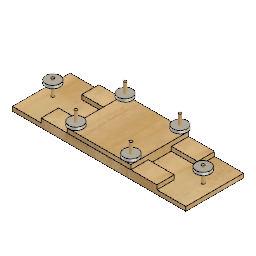
model_X (Autodesk Fusion 360 design; units mm, degrees)
Autodesk Fusion 360 part; units mm, degrees
sketch "Sketch1" plane through (0, 0, 0) normal (0, 0, 1) x (1, 0, 0)
  line L0 (300, 100) -> (-300, 100)
  line L1 (-300, 100) -> (-300, -100)
  line L2 (-300, -100) -> (300, -100)
  line L3 (300, -100) -> (300, 100)
  line L4 (300, 100) -> (-300, -100) construction
  line L5 (-300, 100) -> (300, -100) construction
  circle A0 centre (-260, 0) radius 5
  circle A1 centre (260, 0) radius 5
  line L6 (-200, -100) -> (200, -100)
  line L7 (200, -100) -> (200, -40)
  line L8 (200, -40) -> (-200, -40)
  line L9 (-200, -40) -> (-200, -100)
  line L10 (-200, 100) -> (200, 100)
  line L11 (200, 100) -> (200, 40)
  line L12 (200, 40) -> (-200, 40)
  line L13 (-200, 40) -> (-200, 100)
  circle A2 through (-235, 0, 55) (-272.5, 21.6506, 55) (-272.5, -21.6506, 55)
  circle A3 through (285, 0, 55) (247.5, 21.6506, 55) (247.5, -21.6506, 55)
  dimension "d1" = 600
  dimension "d2" = 200
  dimension "d3" = 40
  dimension "d4" = 40
  dimension "d5" = 10
  dimension "d6" = 10
  dimension "d7" = 400
  dimension "d8" = 60
  dimension "d9" = 400
  dimension "d10" = 60
  dimension "d11" = 100
  dimension "d12" = 100
  measures "d5" diameter of A0
  measures "d6" diameter of A1
  measures "d9" distance of L11 L13
  measures "d10" distance of L0 L12
  measures "d12" distance of L3 L7
extrude "Extrude1" add sketch "Sketch1" along normal blind 15 contours L0 L1 L2 L3 L7 L8 L9 L11 L12 L13 | L0 L10 L11 L12 L13 | L2 L6 L7 L8 L9 | A0 | A1 makes body 1
extrude "Extrude2" add sketch "Sketch1" along normal blind 30 contours L0 L10 L11 L12 L13 | L2 L6 L7 L8 L9 bodies 1
extrude "Extrude3" add sketch "Sketch1" along normal blind 70 contours A0 | A1 bodies 1
ref_plane "WorkPlane1" through (0, 0, 30) normal (0, 0, 1) x (1, 0, 0)
sketch "Sketch2" plane through (0, 0, 30) normal (0, 0, 1) x (1, 0, 0)
  line L0 (110, 39.5) -> (-110, 39.5)
  line L1 (-110, 39.5) -> (-110, -39.5)
  line L2 (-110, -39.5) -> (110, -39.5)
  line L3 (110, -39.5) -> (110, 39.5)
  line L4 (110, 39.5) -> (-110, -39.5) construction
  line L5 (-110, 39.5) -> (110, -39.5) construction
  line L6 (-110, 100) -> (110, 100)
  line L7 (110, 100) -> (110, -100)
  line L8 (110, -100) -> (-110, -100)
  line L9 (-110, -100) -> (-110, 100)
  line L10 (300, 100) -> (-300, 100)
  line L11 (-300, -100) -> (300, -100)
  circle A0 centre (-95, -85) radius 5
  circle A1 centre (95, -85) radius 5
  circle A2 centre (-95, 85) radius 5
  circle A3 centre (95, 85) radius 5
  circle A4 through (120, -85, 25) (82.5, -63.3494, 25) (82.5, -106.6506, 25)
  circle A5 through (-70, -85, 25) (-107.5, -63.3494, 25) (-107.5, -106.6506, 25)
  circle A6 through (-70, 85, 25) (-107.5, 106.6506, 25) (-107.5, 63.3494, 25)
  circle A7 through (120, 85, 25) (82.5, 106.6506, 25) (82.5, 63.3494, 25)
  line L12 (-70, -85) -> (-70, -100) construction
  line L13 (69.9377, -85) -> (70, -100) construction
  line L14 (70, 85) -> (70, 100) construction
  line L15 (-70, 85) -> (-70, 100) construction
  line L16 (70, -100) -> (60, -100) construction
  line L17 (-70, 100) -> (-60, 100) construction
  line L18 (-60, 100) -> (60, 100)
  line L19 (60, 100) -> (60, -100)
  line L20 (60, -100) -> (-60, -100)
  line L21 (-60, -100) -> (-60, 100)
  line L22 (30, 100) -> (-30, 100)
  line L23 (-30, 100) -> (-30, -100)
  line L24 (-30, -100) -> (30, -100)
  line L25 (30, -100) -> (30, 100)
  line L26 (30, 100) -> (-30, -100) construction
  line L27 (-30, 100) -> (30, -100) construction
  dimension "d20" = 220
  dimension "d21" = 79
  dimension "d22" = 220
  dimension "d27" = 10
  dimension "d28" = 15
  dimension "d29" = 15
  dimension "d30" = 10
  dimension "d31" = 10
  dimension "d32" = 10
  dimension "d33" = 15
  dimension "d34" = 15
  dimension "d35" = 15
  dimension "d36" = 15
  dimension "d37" = 15
  dimension "d38" = 15
  dimension "d59" = 10
  dimension "d60" = 10
  dimension "d61" = 120
  dimension "d62" = 200
  dimension "d63" = 60
  measures "d22" distance of L7 L9
  measures "d27" diameter of A0
  measures "d30" diameter of A1
  measures "d31" diameter of A2
  measures "d32" diameter of A3
extrude "Extrude6" add sketch "Sketch2" against normal blind 14 separate body contours L0 L2 L3 L7 L19 | L0 L2 L19 L25 | L0 L2 L23 L25 | L0 L2 L21 L23 | L0 L1 L2 L9 L21 makes body 2
extrude "Extrude4" add sketch "Sketch1" along normal blind 10 separate body contours A2 | A3 in plane through (0, 0, 55) normal (0, 0, 1) makes body 3 at (-264.7538, 2.2158, 55) makes body 4 at (265.8316, 4.4538, 55)
extrude "Extrude7" add sketch "Sketch2" along normal blind 15 contours L0 L2 L3 L7 L19 | L0 L6 L7 L10 L19 | L0 L2 L19 L25 | L0 L6 L10 L18 L19 L25 | L2 L7 L8 L11 L19 | L0 L2 L23 L25 | L0 L6 L10 L18 L22 L23 L25 | L2 L8 L11 L19 L20 L25 | L0 L2 L21 L23 | L0 L6 L10 L18 L21 L23 | L2 L8 L11 L20 L23 L24 L25 | L0 L1 L2 L9 L21 | L0 L6 L9 L10 L21 | L2 L8 L11 L20 L21 L23 | L2 L8 L9 L11 L21 | A0 | A1 | A2 | A3 bodies 2
extrude "Extrude8" add sketch "Sketch2" along normal blind 70 contours A0 | A1 | A2 | A3 bodies 2
extrude "Extrude9" add sketch "Sketch2" along normal blind 10 separate body contours A4 | A5 | A6 | A7 in plane through (0, 0, 55) normal (0, 0, 1) makes body 5 at (92.4105, -86.6853, 55) makes body 6 at (88.6141, 88.0753, 55) makes body 7 at (-97.5895, -86.6853, 55) makes body 8 at (-101.3859, 88.0753, 55)
equation "d4 = d3"
equation "d6 = d5"
equation "d9 = d7"
equation "d10 = d8"
equation "d12 = d11"
equation "d22 = d20"
equation "d33 = d29"
equation "d34 = d28"
equation "d35 = d29"
equation "d36 = d28"
equation "d37 = d29"
equation "d38 = d28"
named bodies: "rolamento1", "rolamento2", "rolamento3", "rolamento4", "rolamento5", "rolamento6"
